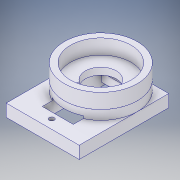
# Autodesk Inventor part: middle
Saved by Autodesk Inventor 2017 (Build 210142000, 142)
## iProperties
Created: 2017-03-11
Part Number: middle
Material: Generic
Document SubType Name: Modeling
Designer: Naga
Density: 1 g/cm^3
Appearance: Cool White
Author: Naga
Autodesk Inventor part; units mm, degrees
ref_plane "YZ Plane" through (0, 0, 0) normal (1, 0, 0) x (0, 1, 0)
ref_plane "XZ Plane" through (0, 0, 0) normal (0, 1, 0) x (-1, 0, 0)
sketch "Sketch1" plane through (0, 0, 0) normal (0, 1, 0) x (-1, 0, 0)
  line L0 (0, 0) -> (29.5, 0)
  line L1 (29.5, 0) -> (29.5, -36.2)
  line L2 (29.5, -36.2) -> (0, -36.2)
  line L3 (0, -36.2) -> (0, 0)
  dimension "d0" = 29.5
  dimension "d1" = 36.2
  constraints: 8 end point, 2 parallel, 1 horizontal, 1 perpendicular
  measures "d0" distance of L1.end L2.end
  measures "d1" distance of L0.end L1.end
extrude "Extrusion1" add sketch "Sketch1" along normal blind 5
sketch "Sketch2" plane through (0, 5, 0) normal (0, 1, 0) x (1, 0, 0)
  line L0 (-29.5, 0) -> (0, 0) projected
  line L1 (-14.75, 0) -> (-14.75, 17.5)
  arc A0 (-18.4298, 18.4481) -> (-11.0702, 18.4481) centre (-14.75, 17.5) ccw
  line L2 (-14.75, 17.5) -> (-14.75, 23.5)
  arc A1 (-11.0702, 18.4481) -> (-18.4298, 18.4481) centre (-14.75, 23.5) ccw
  circle A2 centre (-14.75, 23.5) radius 12.175
  circle A3 centre (-14.75, 23.5) radius 14.75
  dimension "d4" = 17.5
  dimension "d5" = 7.6
  dimension "d6" = 6
  dimension "d7" = 12.5
  dimension "d8" = 24.35
  dimension "d9" = 29.5
  constraints: 4 centre point, 4 coincident, 4 end point, 4 point on circle, 2 vertical, 1 midpoint
  measures "d4" distance of L1.start L1.end
  measures "d5" diameter of A0
  measures "d6" distance of L2.start L2.end
  measures "d7" diameter of A1
  measures "d8" diameter of A2
  measures "d9" diameter of A3
extrude "Extrusion2" add sketch "Sketch2" along normal blind 3.8 contours A2 | A3
sketch "Sketch4" plane through (-14.75, 8.8, -23.5) normal (0, 1, 0) x (1, 0, 0)
  circle A0 centre (0, 0) radius 12.25
  circle A1 centre (0, 0) radius 14.7438
  point P0 (14.75, -23.5)
  dimension "d12" = 24.5
  constraints: 2 centre point, 1 coincident
  measures "d12" diameter of A0
extrude "Extrusion3" add sketch "Sketch4" along normal blind 6
sketch "Sketch5" plane through (-14.75, 8.8, -23.5) normal (0, 1, 0) x (1, 0, 0)
  arc A0 (-3.6798, -5.0519) -> (3.6798, -5.0519) centre (0, -6) ccw projected
  arc A1 (3.6798, -5.0519) -> (-3.6798, -5.0519) centre (0, 0) ccw projected
  point P0 (14.75, -23.5)
extrude "Extrusion4" cut sketch "Sketch5" against normal up to surface (8.8 mm away)
sketch "Sketch6" plane through (0, 0, 0) normal (0, -1, 0) x (1, 0, 0)
  arc A0 (-11.0702, -18.4481) -> (-18.4298, -18.4481) centre (-14.75, -17.5) ccw projected
  arc A1 (-18.4298, -18.4481) -> (-11.0702, -18.4481) centre (-14.75, -23.5) ccw projected
  line L0 (0, 0) -> (-29.5, 0) projected
  line L1 (-29.5, 0) -> (-29.5, -36.2) projected
  line L2 (-29.5, -36.2) -> (0, -36.2) projected
  line L3 (0, -36.2) -> (0, 0) projected
  line L4 (-14.75, 0) -> (-14.75, -36.2)
  line L5 (0, -36.2) -> (0, 0) projected
  line L6 (0, -18.1) -> (-29.5, -18.1)
  line L7 (-21.0275, -1.55) -> (-8.4725, -1.55)
  line L8 (-8.4725, -1.55) -> (-8.4725, -34.65)
  line L9 (-8.4725, -34.65) -> (-21.0275, -34.65)
  line L10 (-21.0275, -34.65) -> (-21.0275, -1.55)
  line L11 (-21.0275, -1.55) -> (-8.4725, -34.65) construction
  line L12 (-8.4725, -1.55) -> (-21.0275, -34.65) construction
  point P0 (-14.75, -18.1)
  dimension "d17" = 12.555
  dimension "d18" = 33.1
  constraints: 16 end point, 7 midpoint, 2 parallel, 1 horizontal, 1 perpendicular
  measures "d17" distance of L8.end L9.end
  measures "d18" distance between parallel lines of L9 L7
extrude "Extrusion5" cut sketch "Sketch6" against normal blind 6 contours A0 L6 L8 L9 L4 A1 | A0 L4 L7 L8 L6 | L4 L9 L10 L6 A0 A1 | A0 L6 L10 L7 L4
ref_plane "Work Plane1" through (0, 1.5, 0) normal (0, -1, 0) x (1, 0, 0)
sketch "Sketch7" plane through (0, 1.5, 0) normal (0, -1, 0) x (1, 0, 0)
  line L0 (-8.4725, -1.55) -> (-8.4725, -34.65) projected
  line L1 (-8.4725, -34.65) -> (-21.0275, -34.65) projected
  line L2 (-21.0275, -1.55) -> (-8.4725, -1.55) projected
  line L3 (-21.0275, -34.65) -> (-21.0275, -1.55) projected
  line L4 (-8.4725, -1.55) -> (-21.0275, -1.55)
  line L5 (-21.0275, -1.55) -> (-21.0275, -6.091)
  line L6 (-21.0275, -6.091) -> (-8.4725, -6.091)
  line L7 (-8.4725, -6.091) -> (-8.4725, -1.55)
  line L8 (-8.4725, -34.65) -> (-21.0201, -34.65)
  line L9 (-21.0201, -34.65) -> (-21.0201, -30.109)
  line L10 (-21.0201, -30.109) -> (-8.4725, -30.109)
  line L11 (-8.4725, -30.109) -> (-8.4725, -34.65)
  line L12 (-14.75, -1.55) -> (-14.7463, -34.65)
  line L13 (-14.75, -1.55) -> (-14.7498, -3.632)
  line L14 (-14.7463, -34.65) -> (-14.7465, -32.568)
  circle A0 centre (-14.7498, -3.632) radius 1
  circle A1 centre (-14.7465, -32.568) radius 1
  point P0 (0, 0)
  dimension "d22" = 4.541
  dimension "d23" = 12.555
  dimension "d24" = 4.541
  dimension "d25" = 12.5476
  dimension "d26" = 2.082
  dimension "d27" = 0
  dimension "d28" = 2.082
  dimension "d29" = 0
  dimension "d30" = 2
  dimension "d31" = 2
  constraints: 22 end point, 4 parallel, 2 centre point, 2 coincident, 2 horizontal, 2 midpoint, 2 perpendicular
  measures "d22" distance of L4.end L5.end
  measures "d23" distance of L5.end L6.end
  measures "d24" distance of L8.end L9.end
  measures "d25" distance of L9.end L10.end
  measures "d26" distance of L12.start L13.end
  measures "d27" distance between parallel lines of L12 L13
  measures "d28" distance of L12.end L14.end
  measures "d29" distance between parallel lines of L12 L14
  measures "d30" diameter of A0
  measures "d31" diameter of A1
extrude "Extrusion6" add sketch "Sketch7" against normal up to surface (3.5 mm away) contours L0 L6 L12 A0 L2 | L12 A0 L6 L3 L2 | L0 L1 L12 A1 L10 | L12 A1 L1 L9 L10
body "Solid1"
